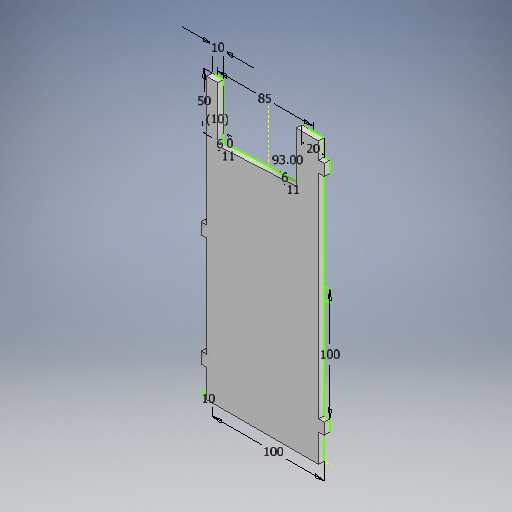
# Autodesk Inventor part: Lifting Sections leftt
Saved by Autodesk Inventor 2025.3 (Build 293356000, 356)
## iProperties
Created: 2026-04-06
Part Number: Lifting Sections leftt
Material: Generic
Document SubType Name: Modeling
Designer: user
Density: 1 g/cm^3
Appearance: Default
Author: user
Autodesk Inventor part; units mm, degrees
ref_plane "YZ Plane" through (0, 0, 0) normal (1, 0, 0) x (0, 1, 0)
ref_plane "XZ Plane" through (0, 0, 0) normal (0, 1, 0) x (-1, 0, 0)
ref_plane "XY Plane" through (0, 0, 0) normal (0, 0, 1) x (1, 0, 0)
sketch "Sketch1" plane through (0, 0, 0) normal (0, 0, 1) x (1, 0, 0)
  line L0 (-68.6002, -120.3249) -> (31.3998, -120.3249)
  line L1 (31.3998, -120.3249) -> (31.3998, 129.6751)
  line L2 (31.3998, 129.6751) -> (11.3998, 129.6751)
  line L3 (11.3998, 129.6751) -> (11.3998, 84.6751)
  line L4 (11.3998, 84.6751) -> (-58.6002, 81.0066)
  line L5 (-68.6002, -120.3249) -> (-68.6002, 77.725)
  line L6 (-68.6002, 77.725) -> (-68.6002, 129.6751)
  line L7 (-68.6002, 129.6751) -> (-58.6002, 129.6751)
  line L8 (-58.6002, 129.6751) -> (-58.6002, 81.0066)
  line L9 (31.3998, -120.3249) -> (41.3973, -120.3249) construction
  line L10 (31.3998, 4.6751) -> (-68.6002, 4.6751) construction
  line L11 (31.3998, 4.6751) -> (36.4024, 4.6751)
  line L12 (36.4024, 14.8241) -> (31.3973, 14.8241)
  line L13 (31.3973, 14.8241) -> (31.3998, 4.6751)
  line L14 (-68.6002, 129.6751) -> (-68.6002, 79.6751)
  line L15 (-68.6002, 79.6751) -> (31.3998, 79.6751) construction
  line L16 (36.3973, 114.8241) -> (31.3973, 114.8241)
  line L17 (31.3973, 104.7241) -> (36.3973, 104.7241)
  line L18 (36.3973, -85.1759) -> (31.3973, -85.1759)
  line L19 (31.3973, -95.2759) -> (36.3973, -95.2759)
  line L20 (36.4024, 14.8241) -> (31.4024, 14.8241)
  line L21 (31.4024, 4.7241) -> (36.4024, 4.7241)
  line L22 (-18.6002, -120.3249) -> (-18.6002, 129.7241) construction
  line L23 (-73.6027, 14.8241) -> (-68.5976, 14.8241)
  line L24 (-73.6027, 14.8241) -> (-68.6027, 14.8241)
  line L25 (-68.6002, 4.6751) -> (-73.6027, 4.6751)
  line L26 (-68.6027, 4.7241) -> (-73.6027, 4.7241)
  line L27 (-73.6027, 4.6751) -> (-73.6027, 14.8241)
  line L28 (-73.6027, 4.7241) -> (-73.6027, 14.8241)
  line L29 (-73.5976, -85.1759) -> (-68.5976, -85.1759)
  line L30 (-73.5976, -95.2759) -> (-73.5976, -85.1759)
  line L31 (-68.5976, -95.2759) -> (-73.5976, -95.2759)
  line L32 (-68.6002, -120.3249) -> (-78.6002, -120.3249)
  line L33 (-58.6002, 81.0066) -> (-68.6002, 81.0556) construction
  line L34 (36.4024, 14.8241) -> (36.4024, 4.7241)
  line L35 (36.3973, 114.8241) -> (36.3973, 104.7241)
  line L36 (36.3973, -85.1759) -> (36.3973, -95.2759)
  line L37 (11.2345, 78.6582) -> (0.2496, 78.0825)
  line L38 (0.2496, 78.0825) -> (-0.0644, 84.0743)
  line L39 (-0.0644, 84.0743) -> (10.9205, 84.65)
  line L40 (10.9205, 84.65) -> (11.2345, 78.6582)
  line L41 (-57.9849, 81.0388) -> (10.9205, 84.65)
  line L42 (-57.6709, 75.047) -> (-57.9849, 81.0388)
  line L43 (-46.686, 75.6227) -> (-57.6709, 75.047)
  line L44 (-47, 81.6145) -> (-46.686, 75.6227)
  point P0 (0, 0)
  point P1 (21.3998, 129.6751)
  point P2 (-63.6002, 129.6751)
  point P3 (-68.6002, 14.8241)
  point P4 (-68.6002, 4.6751)
  point P5 (-68.6002, -85.1759)
  point P6 (-68.6002, -95.2759)
  point P7 (31.3998, -95.2759)
  point P8 (31.3998, -85.1759)
  point P9 (36.3973, 4.7241)
  point P10 (36.4024, 14.8241)
  point P11 (31.3998, 14.8241)
  point P12 (31.3998, 104.7241)
  point P13 (31.3998, 114.8241)
  dimension "d0" = 100
  dimension "d2" = 20
  dimension "d4" = 93
  dimension "d5" = 10
  dimension "d6" = 85
  dimension "d10" = 50
  dimension "d12" = 100
  dimension "d13" = 10
  dimension "d33" = 11
  dimension "d34" = 6
  dimension "d35" = 10
  dimension "d36" = 11
  dimension "d37" = 6
  dimension "d43" = 0
  constraints: 90 end point, 12 symmetric about line, 6 parallel, 6 perpendicular, 6 point on line, 6 vertical, 5 horizontal, 4 midpoint, 2 collinear
  measures "d0" distance of L0.start L1.start
  measures "d2" distance of L1.end L3.start
  measures "d4" angle of L3 L4
  measures "d5" distance of L6.end L7.end
  measures "d6" distance of point (21.4, 129.675) point (-63.6, 129.675)
  measures "d10" distance of L6.end L15.start
  measures "d12" distance of L12.start L18.start
  measures "d13" distance of L0.start L32.end
  measures "d33" distance of L37.start L38.start
  measures "d34" distance of L38.start L39.start
  measures "d35" distance between parallel lines of L14 L8
  measures "d36" distance of L44.end L43.end
  measures "d37" distance of L41.start L43.end
  measures "d43" distance between parallel lines of L41 L4
extrude "Extrusion1" add sketch "Sketch1" along normal blind 5
body "Solid1"
